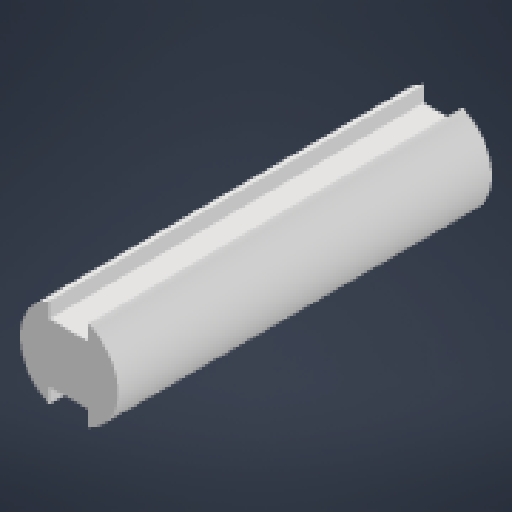
# Autodesk Inventor part: long_axel
Saved by Autodesk Inventor 2026 (Build 300175050, 175E)
## iProperties
Created: 2026-04-30
Part Number: long_axel
Material: Generic
Document SubType Name: Modeling
Designer: sniel
Density: 1 g/cm^3
Appearance: Default
Author: sniel
Autodesk Inventor part; units mm, degrees
ref_plane "YZ Plane" through (0, 0, 0) normal (1, 0, 0) x (0, 1, 0)
ref_plane "XZ Plane" through (0, 0, 0) normal (0, 1, 0) x (-1, 0, 0)
ref_plane "XY Plane" through (0, 0, 0) normal (0, 0, 1) x (1, 0, 0)
sketch "Sketch1" plane through (0, 0, 0) normal (0, 0, 1) x (1, 0, 0)
  circle A0 centre (0, 0) radius 3.925
  line L0 (-1.575, 5.5) -> (1.575, 5.5)
  line L1 (1.575, 5.5) -> (1.575, 2.35)
  line L2 (1.575, 2.35) -> (-1.575, 2.35)
  line L3 (-1.575, 2.35) -> (-1.575, 5.5)
  line L4 (-1.575, 5.5) -> (1.575, 2.35) construction
  line L5 (1.575, 5.5) -> (-1.575, 2.35) construction
  line L6 (-1.575, -5.5) -> (1.575, -5.5)
  line L7 (1.575, -5.5) -> (1.575, -2.35)
  line L8 (1.575, -2.35) -> (-1.575, -2.35)
  line L9 (-1.575, -2.35) -> (-1.575, -5.5)
  line L10 (-1.575, -5.5) -> (1.575, -2.35) construction
  line L11 (1.575, -5.5) -> (-1.575, -2.35) construction
  point P0 (0, 3.925)
  point P1 (0, -3.925)
  point P2 (-1.575, 3.5951)
  point P3 (-1.575, -3.5951)
  point P4 (1.575, -3.5951)
  point P5 (1.575, 3.5951)
  dimension "d0" = 7.85
  dimension "d1" = 3.15
  dimension "d2" = 3.15
  dimension "d3" = 3.15
  dimension "d4" = 3.15
  constraints: 24 end point, 4 midpoint, 4 parallel, 2 horizontal, 2 perpendicular, 2 point on circle, 1 centre point, 1 coincident
  measures "d0" diameter of A0
  measures "d1" distance of L1.end L2.end
  measures "d2" distance of L0.end L1.end
  measures "d3" distance of L8.end L7.end
  measures "d4" distance of L7.end L6.end
extrude "Extrusion1" add sketch "Sketch1" along normal blind 30 contours A0 L7 L8 L9 L3 L2 L1
body "Solid1"
